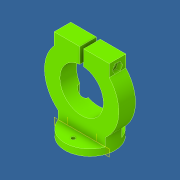
# Autodesk Inventor part: GripperMountProxxon
Saved by Autodesk Inventor 2016 (Build 200138000, 138)
## iProperties
Created: 2015-09-10
Part Number: GripperMountProxxon
Material: ABS-Kunststoff
Document SubType Name: Modeling
Designer: 4ndreas
Density: 1.06 g/cm^3
Appearance: Glatt - grün
Mass: 7.0775 g
Surface Area: 34.9537 cm^2
Volume: 6.67689 cm^3
Author: 4ndreas
Autodesk Inventor part; units mm, degrees
ref_plane "YZ Plane" through (0, 0, 0) normal (1, 0, 0) x (0, 1, 0)
ref_plane "XZ Plane" through (0, 0, 0) normal (0, 1, 0) x (-1, 0, 0)
ref_plane "XY Plane" through (0, 0, 0) normal (0, 0, 1) x (1, 0, 0)
sketch "Skizze1" plane through (0, 0, 0) normal (0, 0, 1) x (1, 0, 0)
  circle A0 centre (-11.2583, 6.5) radius 1.5 projected
  circle A1 centre (-11.2583, -6.5) radius 1.5 projected
  circle A2 centre (0, -13) radius 1.5 projected
  circle A3 centre (11.2583, -6.5) radius 1.5 projected
  circle A4 centre (11.2583, 6.5) radius 1.5 projected
  circle A5 centre (0, 13) radius 1.5 projected
  arc A6 (14.3761, 1.8914) -> (11.9393, 3.5783) centre (12.3932, 1.6305) ccw projected
  arc A7 (14.3761, -1.8914) -> (14.3761, 1.8914) centre (0, 0) ccw projected
  arc A8 (11.9393, -3.5783) -> (14.3761, -1.8914) centre (12.3932, -1.6305) ccw projected
  arc A9 (11.9393, -3.5783) -> (9.0685, -8.5505) centre (11.2583, -6.5) ccw projected
  arc A10 (8.826, -11.5044) -> (9.0685, -8.5505) centre (7.6087, -9.9176) ccw projected
  arc A11 (5.5501, -13.3958) -> (8.826, -11.5044) centre (0, 0) ccw projected
  arc A12 (2.8707, -12.1288) -> (5.5501, -13.3958) centre (4.7846, -11.5481) ccw projected
  arc A13 (2.8707, -12.1288) -> (-2.8707, -12.1288) centre (0, -13) ccw projected
  arc A14 (-5.5501, -13.3958) -> (-2.8707, -12.1288) centre (-4.7846, -11.5481) ccw projected
  arc A15 (-8.826, -11.5044) -> (-5.5501, -13.3958) centre (0, 0) ccw projected
  arc A16 (-9.0685, -8.5505) -> (-8.826, -11.5044) centre (-7.6087, -9.9176) ccw projected
  arc A17 (-9.0685, -8.5505) -> (-11.9393, -3.5783) centre (-11.2583, -6.5) ccw projected
  arc A18 (-14.3761, -1.8914) -> (-11.9393, -3.5783) centre (-12.3932, -1.6305) ccw projected
  arc A19 (-14.3761, 1.8914) -> (-14.3761, -1.8914) centre (0, 0) ccw projected
  arc A20 (-11.9393, 3.5783) -> (-14.3761, 1.8914) centre (-12.3932, 1.6305) ccw projected
  arc A21 (-11.9393, 3.5783) -> (-9.0685, 8.5505) centre (-11.2583, 6.5) ccw projected
  arc A22 (-8.826, 11.5044) -> (-9.0685, 8.5505) centre (-7.6087, 9.9176) ccw projected
  arc A23 (-5.5501, 13.3958) -> (-8.826, 11.5044) centre (0, 0) ccw projected
  arc A24 (-2.8707, 12.1288) -> (-5.5501, 13.3958) centre (-4.7846, 11.5481) ccw projected
  arc A25 (-2.8707, 12.1288) -> (2.8707, 12.1288) centre (0, 13) ccw projected
  arc A26 (5.5501, 13.3958) -> (2.8707, 12.1288) centre (4.7846, 11.5481) ccw projected
  arc A27 (8.826, 11.5044) -> (5.5501, 13.3958) centre (0, 0) ccw projected
  arc A28 (9.0685, 8.5505) -> (8.826, 11.5044) centre (7.6087, 9.9176) ccw projected
  arc A29 (9.0685, 8.5505) -> (11.9393, 3.5783) centre (11.2583, 6.5) ccw projected
  circle A30 centre (0, 0) radius 17.5 projected
  circle A31 centre (0, 0) radius 19.5
  point P0 (0, 0)
  dimension "d0" = 39
  constraints: 1 centre point, 1 coincident
  measures "d0" diameter of A31
extrude "Extrusion1" add sketch "Skizze1" along normal blind 5 contours A7 A8 A9 A10 A11 A12 A13 A14 A15 A16 A17 A18 A19 A20 A21 A22 A23 A24 A25 A26 A27 A28 A29 A6 | A30 | A31
ref_plane "Arbeitsebene1" through (11.2583, -6.5, 0) normal (0, -1, 0) x (0, 0, 1)
sketch "Skizze7" plane through (11.2583, -6.5, 0) normal (0, -1, 0) x (0, 0, 1)
  line L0 (0, 21.0167) -> (5, 21.0167) projected
  line L1 (5, 21.0167) -> (5, 1.5) projected
  line L2 (5, 1.5) -> (0, 1.5) projected
  line L3 (0, 1.5) -> (0, 21.0167) projected
  line L4 (5, -7.1264) -> (0, -7.1264) projected
  line L5 (0, -7.1264) -> (0, -1.5) projected
  line L6 (0, -1.5) -> (5, -1.5) projected
  line L7 (5, -1.5) -> (5, -7.1264) projected
  line L8 (0, 29.6431) -> (5, 29.6431) projected
  line L9 (5, 29.6431) -> (5, 24.0167) projected
  line L10 (5, 24.0167) -> (0, 24.0167) projected
  line L11 (0, 24.0167) -> (0, 29.6431) projected
  line L12 (5, 1.5) -> (17, 1.5)
  line L13 (17, 1.5) -> (17, 21.0167)
  line L14 (17, 21.0167) -> (5, 21.0167)
  line L15 (5, 21.0167) -> (5, 1.5)
  arc A0 (50.9337, 12.7583) -> (50.9337, 9.7583) centre (34, 11.2583) ccw
  arc A1 (62.9612, 12.7583) -> (62.9612, 9.7583) centre (34, 11.2583) ccw
  line L16 (50.9337, 9.7583) -> (62.9612, 9.7583)
  line L17 (50.9337, 12.7583) -> (62.9612, 12.7583)
  line L18 (34, 11.2583) -> (5, 11.2583) construction
  line L19 (5, -7.1264) -> (11.5723, -7.1264)
  line L20 (5, 29.6431) -> (11.5723, 29.6431)
  line L21 (5, -7.1264) -> (5, 29.6431)
  point P0 (0, 11.2583)
  dimension "d26" = 3
  dimension "d27" = 17
  dimension "d28" = 12
  constraints: 20 end point, 6 point on circle, 4 horizontal, 3 parallel, 2 centre point, 2 perpendicular, 2 tangent, 1 coincident, 1 collinear, 1 midpoint, 1 vertical, 1 other
  measures "d26" distance between parallel lines of L17 L16
  measures "d27" radius of A0
  measures "d28" distance between parallel lines of L1 L13
extrude "Extrusion6" add sketch "Skizze7" against normal blind 13 contours L14 A1 L1 | L21 L9 L20 A1 L14 | A1 L12 L1 | A1 L14 L13 L12 | A1 L17 A0 L13 L14 | L12 A1 L19 L7 L21 | L12 L13 A0 L16 A1
sketch "Skizze8" plane through (1.5, -6.5, 50.9337) normal (-1, 0, 0) x (0, 0, 1)
  line L0 (12.0275, 0) -> (0, 0) projected
  line L1 (0, 0) -> (0, 13) projected
  line L2 (0, 13) -> (12.0275, 13) projected
  line L3 (12.0275, 13) -> (12.0275, 0) projected
  line L4 (-45.9337, 25.9422) -> (-45.9337, 19.5) projected
  line L5 (-45.9337, 19.5) -> (-45.9337, 13) projected
  line L6 (-45.9337, 13) -> (-33.8674, 13) projected
  line L7 (-33.8674, 13) -> (-33.8674, 0) projected
  line L8 (-33.8674, 0) -> (-45.9337, 0) projected
  line L9 (-45.9337, 0) -> (-45.9337, -6.5) projected
  line L10 (-45.9337, -6.5) -> (-50.9337, -6.5) projected
  line L11 (-50.9337, -6.5) -> (-50.9337, 19.5) projected
  line L12 (-50.9337, 19.5) -> (-50.9337, 25.9422) projected
  line L13 (-50.9337, 25.9422) -> (-45.9337, 25.9422) projected
  line L14 (-45.9337, 19.5) -> (-50.9337, 19.5) projected
  line L15 (-45.9337, -6.5) -> (-45.9337, -12.9422) projected
  line L16 (-45.9337, -12.9422) -> (-50.9337, -12.9422) projected
  line L17 (-50.9337, -12.9422) -> (-50.9337, -6.5) projected
  point P0 (-50.9337, 6.5)
extrude "Extrusion7" add sketch "Skizze8" against normal blind 20 contours L0 L1 L2 L3
sketch "Skizze9" plane through (-1.5, -6.5, 62.9612) normal (1, 0, 0) x (0, 0, -1)
  line L0 (12.0275, 0) -> (0, 0) projected
  line L1 (0, 0) -> (0, 13) projected
  line L2 (0, 13) -> (12.0275, 13) projected
  line L3 (12.0275, 13) -> (12.0275, 0) projected
  line L4 (57.9612, -12.9422) -> (57.9612, -6.5) projected
  line L5 (57.9612, -6.5) -> (57.9612, 0) projected
  line L6 (57.9612, 0) -> (45.8949, 0) projected
  line L7 (45.8949, 0) -> (45.8949, 13) projected
  line L8 (45.8949, 13) -> (57.9612, 13) projected
  line L9 (57.9612, 13) -> (57.9612, 19.5) projected
  line L10 (57.9612, 19.5) -> (62.9612, 19.5) projected
  line L11 (62.9612, 19.5) -> (62.9612, -6.5) projected
  line L12 (62.9612, -6.5) -> (62.9612, -12.9422) projected
  line L13 (62.9612, -12.9422) -> (57.9612, -12.9422) projected
  line L14 (57.9612, -6.5) -> (62.9612, -6.5) projected
  line L15 (57.9612, 19.5) -> (57.9612, 25.9422) projected
  line L16 (57.9612, 25.9422) -> (62.9612, 25.9422) projected
  line L17 (62.9612, 25.9422) -> (62.9612, 19.5) projected
  point P0 (62.9612, 6.5)
extrude "Extrusion8" add sketch "Skizze9" against normal blind 20 contours L0 L1 L2 L3
sketch "Skizze10" plane through (0, 0, 5) normal (0, 0, 1) x (1, 0, 0)
  circle A0 centre (0, 13) radius 1.5 projected
  circle A1 centre (11.2583, 6.5) radius 1.5 projected
  circle A2 centre (11.2583, -6.5) radius 1.5 projected
  circle A3 centre (0, -13) radius 1.5 projected
  circle A4 centre (-11.2583, -6.5) radius 1.5 projected
  circle A5 centre (-11.2583, 6.5) radius 1.5 projected
  circle A6 centre (0, 0) radius 19.5 projected
  circle A7 centre (11.2583, 6.5) radius 3.5
  circle A8 centre (-11.2583, 6.5) radius 3.5
  line L0 (12.7583, 6.5) -> (9.7583, 6.5) projected
  point P0 (0, 0)
  dimension "d35" = 7
  constraints: 2 centre point, 2 coincident, 1 equal radius, 1 midpoint
  measures "d35" diameter of A7
extrude "Extrusion9" cut sketch "Skizze10" along normal blind 20 contours L0 A1 | A1 L0 | A5 | A7 | A8
sketch "Skizze11" plane through (0, 0, 0) normal (0, 0, -1) x (-1, 0, 0)
  circle A0 centre (0, 13) radius 1.5 projected
  circle A1 centre (-11.2583, 6.5) radius 1.5 projected
  circle A2 centre (-11.2583, -6.5) radius 1.5 projected
  circle A3 centre (0, -13) radius 1.5 projected
  circle A4 centre (11.2583, -6.5) radius 1.5 projected
  circle A5 centre (11.2583, 6.5) radius 1.5 projected
  circle A6 centre (0, 0) radius 19.5 projected
  point P0 (0, 0)
extrude "Extrusion10" add sketch "Skizze11" against normal up to surface (5 mm away) contours A0 | A2 | A4
sketch "Skizze13" plane through (-21.5, -6.5, 62.9612) normal (-1, 0, 0) x (0, 0, 1)
  line L0 (-12.0275, 0) -> (0, 0) projected
  line L1 (-12.0275, 0) -> (-12.0275, 13) projected
  line L2 (0, 13) -> (-12.0275, 13) projected
  line L3 (0, 0) -> (0, 13) projected
  line L4 (-12.0275, 0) -> (0, 0)
  line L5 (0, 0) -> (0, 13)
  line L6 (0, 13) -> (-12.0275, 13)
  line L7 (-12.0275, 13) -> (-12.0275, 0)
  line L8 (-12.0275, 0) -> (0, 13) construction
  line L9 (0, 0) -> (-12.0275, 13) construction
  point P0 (-62.9612, 6.5)
  point P1 (-6.0137, 6.5)
  constraints: 12 end point, 2 collinear, 2 midpoint, 2 parallel, 1 horizontal, 1 perpendicular
hole "Bohrung2" at (-21.5, 0, 56.9474) direction (1, 0, 0) diameter 4.2 end through all
sketch "Skizze14" plane through (-21.5, -6.5, 62.9612) normal (-1, 0, 0) x (0, 0, 1)
  circle A0 centre (-6.0137, 6.5) radius 2.1 projected
  line L0 (-9.4997, 0) -> (-9.4997, 13) projected
  line L1 (-9.4997, 0) -> (0, 0) projected
  line L2 (0, 0) -> (0, 13) projected
  line L3 (0, 13) -> (-9.4997, 13) projected
  circle A1 centre (-6.0137, 6.5) radius 4.5
  point P0 (-62.9612, 6.5)
  dimension "d47" = 9
  constraints: 1 centre point, 1 coincident
  measures "d47" diameter of A1
extrude "Extrusion11" cut sketch "Skizze14" along normal blind 2 contours A0 | A1 L0 | L0 A1
sketch "Skizze15" plane through (21.5, -6.5, 50.9337) normal (1, 0, 0) x (0, 0, -1)
  circle A0 centre (-6.0137, 6.5) radius 2.1 projected
  line L0 (-2.5278, 13) -> (-2.5278, 0) projected
  line L1 (-2.5278, 13) -> (-12.0275, 13) projected
  line L2 (-12.0275, 13) -> (-12.0275, 0) projected
  line L3 (-12.0275, 0) -> (-2.5278, 0) projected
  line L4 (-6.0137, 10.5415) -> (-2.5137, 8.5207)
  line L5 (-2.5137, 8.5207) -> (-2.5137, 4.4793)
  line L6 (-2.5137, 4.4793) -> (-6.0137, 2.4585)
  line L7 (-6.0137, 2.4585) -> (-9.5137, 4.4793)
  line L8 (-9.5137, 4.4793) -> (-9.5137, 8.5207)
  line L9 (-9.5137, 8.5207) -> (-6.0137, 10.5415)
  line L10 (-12.0275, 13) -> (-12.0275, 0) projected
  point P0 (50.9337, 6.5)
  dimension "d50" = 7
  constraints: 12 end point, 1 coincident, 1 parallel, 13 other
  measures "d50" distance between parallel lines of L8 L5
extrude "Extrusion12" cut sketch "Skizze15" along normal mid plane 7 contours A0 | L4 L5 L6 L0 | L0 L6 L7 L8 L9 L4
sketch "Skizze16" plane through (0, 0, 5) normal (0, 0, 1) x (1, 0, 0)
  line L0 (-18.3848, -6.5) -> (-18.3848, 6.5) projected
  arc A0 (-18.3848, 6.5) -> (-18.3848, -6.5) centre (0, 0) ccw projected
  line L1 (18.3848, 6.5) -> (18.3848, -6.5) projected
  arc A1 (18.3848, -6.5) -> (18.3848, 6.5) centre (0, 0) ccw projected
  point P0 (0, 0)
extrude "Extrusion13" add sketch "Skizze16" along normal blind 10
sketch "Skizze2" plane through (0, 0, 5) normal (0, 0, 1) x (1, 0, 0)
  circle A0 centre (0, 0) radius 7.5
  dimension "d3" = 15
  dimension "d20" = 7
  dimension "d8" = 7
  constraints: 12 end point, 1 coincident, 1 vertical, 13 other
sketch "Skizze4" plane through (0, 0, 10) normal (0, 0, 1) x (1, 0, 0)
  point P0 (0, 0)
sketch "Skizze5" plane through (0, 0, 3) normal (0, 0, -1) x (-1, 0, 0)
  circle A0 centre (0, 0) radius 2 projected
  circle A1 centre (0, 0) radius 2 projected
